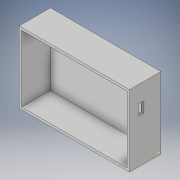
# Autodesk Inventor part: finalCase
Saved by Autodesk Inventor 2018.3 (Build 223284000, 284)
## iProperties
Created: 2019-04-19
Part Number: finalCase
Material: Generic
Document SubType Name: Modeling
Designer: Carlos Lopez
Density: 1 g/cm^3
Appearance: Default
Author: Carlos Lopez
Autodesk Inventor part; units mm, degrees
ref_plane "YZ Plane" through (0, 0, 0) normal (1, 0, 0) x (0, 1, 0)
ref_plane "XZ Plane" through (0, 0, 0) normal (0, 1, 0) x (-1, 0, 0)
ref_plane "XY Plane" through (0, 0, 0) normal (0, 0, 1) x (1, 0, 0)
sketch "Sketch1" plane through (0, 0, 0) normal (0, 0, 1) x (1, 0, 0)
  line L0 (0, 0) -> (83.9978, 0)
  line L1 (83.9978, 0) -> (83.9978, 52.9999)
  line L2 (83.9978, 52.9999) -> (0, 52.9999)
  line L3 (0, 52.9999) -> (0, 0)
  dimension "d0" = 83.9978
  dimension "d1" = 52.9999
  constraints: 8 end point, 2 parallel, 1 horizontal, 1 perpendicular
  measures "d0" distance of L2.end L1.end
  measures "d1" distance of L1.end L0.end
extrude "Extrusion1" add sketch "Sketch1" along normal blind 22.9997
shell "Shell1" thickness 1.9812 outward yes removed faces 1 at (55.9985, 17.6666, 22.9997)
sketch "Sketch2" plane through (85.979, -1.9812, -1.9812) normal (1, 0, 0) x (0, 0, -1)
  point P0 (-1.9812, 1.9812)
sketch "Sketch3" plane through (85.979, -1.9812, -1.9812) normal (1, 0, 0) x (0, 0, -1)
  line L0 (-13.7922, 43.5102) -> (-17.78, 43.5102)
  line L1 (-17.78, 43.5102) -> (-17.78, 35.0012)
  line L2 (-17.78, 35.0012) -> (-13.7922, 35.0012)
  line L3 (-13.7922, 35.0012) -> (-13.7922, 43.5102)
  point P0 (-1.9812, 1.9812)
  dimension "d5" = 3.9878
  dimension "d6" = 8.509
  constraints: 8 end point, 2 parallel, 1 horizontal, 1 perpendicular
  measures "d5" distance of L2.end L1.end
  measures "d6" distance of L1.end L0.end
extrude "Extrusion2" cut sketch "Sketch3" against normal blind 22.9997
body "Solid1"
